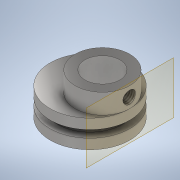
# Autodesk Inventor part: Part17
Saved by Autodesk Inventor 2020 (Build 240168000, 168)
## iProperties
Created: 2021-10-25
Part Number: Part17
Material: Steel, Mild
Document SubType Name: Modeling
Designer: simon.erikssonwestl
Density: 7.85 g/cm^3
Appearance: Semi-Polished
Author: simon.erikssonwestl
Autodesk Inventor part; units mm, degrees
ref_plane "XZ Plane" through (0, 0, 0) normal (0, 1, 0) x (-1, 0, 0)
ref_plane "XY Plane" through (0, 0, 0) normal (0, 0, 1) x (1, 0, 0)
sketch "Sketch1" plane through (0, 0, 0) normal (0, 1, 0) x (-1, 0, 0)
  circle A0 centre (0, 0) radius 8
  dimension "d0" = 16
  constraints: 1 centre point, 1 coincident
  measures "d0" diameter of A0
extrude "Extrusion1" add sketch "Sketch1" along normal blind 2
sketch "Sketch2" plane through (0, 2, 0) normal (0, 1, 0) x (1, 0, 0)
  circle A0 centre (0, 0) radius 6.5
  dimension "d3" = 13
  constraints: 1 centre point, 1 coincident
  measures "d3" diameter of A0
extrude "Extrusion2" add sketch "Sketch2" along normal blind 1.5
sketch "Sketch3" plane through (0, 3.5, 0) normal (0, 1, 0) x (1, 0, 0)
  circle A0 centre (0, 0) radius 8
  dimension "d6" = 16
  constraints: 1 centre point, 1 coincident
  measures "d6" diameter of A0
extrude "Extrusion3" add sketch "Sketch3" along normal blind 2
sketch "Sketch4" plane through (0, 5.5, 0) normal (0, 1, 0) x (1, 0, 0)
  circle A0 centre (2.5, 0) radius 5.5
  circle A1 centre (0, 0) radius 8 projected
  dimension "d9" = 11
  constraints: 1 centre point, 1 tangent
  measures "d9" diameter of A0
extrude "Extrusion4" add sketch "Sketch4" along normal blind 4 contours A0
ref_plane "Work Plane1" through (8, 5.5, 0) normal (1, 0, 0) x (0, 1, 0)
sketch "Sketch5" plane through (8, 5.5, 0) normal (1, 0, 0) x (0, 1, 0)
  line L0 (4, -5.5) -> (4, 5.5) projected
  point P0 (-5.5, 0)
  point P1 (2, 0)
  dimension "d12" = 2
  measures "d12" distance from line of L0 point (2, 0)
hole "Hole1" at (8, 7.5, 0) direction (-1, 0, 0) diameter 2.5 depth 2.15 tip angle 118
thread "Thread1" size "M2.5x0.45" class "6H" standard "ANSI Metric M Profile" length 5.5
sketch "Sketch6" plane through (2.5, 9.5, 0) normal (0, 1, 0) x (1, 0, 0)
  point P0 (-2.5, 0)
  point P1 (0, 0)
hole "Hole2" at (2.5, 9.5, 0) direction (0, -1, 0) diameter 7 end through all
body "Solid1"
